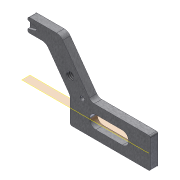
# Autodesk Inventor part: J002859
Saved by Autodesk Inventor 2012 SP2 (Build 160219200, 219)
## iProperties
Created: 2010-10-20
Part Number: J002859
Document SubType Name: Modeling
Designer: D Flickinger
Density: 8 g/cm^3
Material: STAINLESS STEEL, 303
Mass: 13.7432 g
Surface Area: 17.392 cm^2
Volume: 1.7179 cm^3
Description: MPS H Bar Clamp Bottom
Project: P-194005
Vendor: HHMI: JFRC - ID&F
d0: 1.150 in
d1: 1.200 in
d2: 0.575 in
d129: 0.00 deg
d132: 0.750 in
d136: 1.000 in
d137: 118.00 deg
d19: 0.125 in
d20: 0.00 deg
d21: 0.125 in
d22: 0.063 in
d23: 0.050 in
d24: 0.040 in
d25: 0.00 deg
d66: 0.125 in
d191: 0.000 in
ALTERED ITEM DESCRIPTION: N/A
ALTERED ITEM PART NUMBER: N/A
ALTERED ITEM VENDOR: N/A
DESIGN DEPARTMENT: HHMI: JFRC - ID&F
LAB/DEPT: SVOBODA (LAB)
REQUESTING SCIENTIST: PERON, SIMON
SPECIAL FINISH: NONE
SURFACE ROUGHNESS: 63 Ra
Revision Number: -
Autodesk Inventor part; units mm, degrees
ref_plane "YZ Plane" through (0, 0, 0) normal (1, 0, 0) x (0, 1, 0)
sketch "Sketch1" plane through (0, 0, 0) normal (0, 0, 1) x (1, 0, 0)
  line L0 (-20.447, 0) -> (20.447, 0) projected
  line L1 (0, -17.526) -> (0, 25.146) projected
  line L2 (14.605, -11.43) -> (-14.605, -11.43)
  line L3 (-14.605, -11.43) -> (-14.605, 19.05)
  line L4 (-14.605, 19.05) -> (14.605, 19.05)
  line L5 (14.605, 19.05) -> (14.605, -11.43)
  line L6 (-14.605, 16.6688) -> (-14.605, 19.05)
  point P0 (0, 0)
  dimension "d0" = 29.21
  dimension "d1" = 30.48
  dimension "d2" = 14.605
  dimension "d232" = 19.05
  constraints: 10 end point, 2 parallel, 1 collinear, 1 horizontal, 1 perpendicular, 1 point on line
  measures "d0" distance of L3.end L4.end
  measures "d1" distance of L2.end L3.end
  measures "d2" distance between parallel lines of L1 L3
  measures "d232" distance between parallel lines of L0 L4
extrude "Extrusion2" add sketch "Sketch1" along normal blind 3.175
sketch "Sketch2" plane through (0, 0, 3.175) normal (0, 0, 1) x (1, 0, 0)
  line L0 (-14.605, -11.43) -> (-14.605, 19.05) projected
  line L1 (-14.605, 17.78) -> (-11.43, 16.9862)
  line L2 (-11.43, 16.9862) -> (-11.43, 15.3987)
  line L3 (-11.43, 15.3987) -> (-14.605, 14.605)
  line L4 (-14.605, 17.78) -> (-14.605, 14.605)
  line L5 (-14.605, 17.78) -> (-14.605, 19.05)
  arc A0 (-11.43, 15.3987) -> (-11.43, 16.9862) centre (-11.6284, 16.1925) ccw
  point P0 (0, 0)
  dimension "d21" = 3.175
  dimension "d22" = 1.5875
  dimension "d23" = 1.27
  dimension "d66" = 3.175
  constraints: 10 end point, 2 collinear, 2 point on circle, 2 point on line, 1 centre point, 1 equal length, 1 parallel, 1 tangent
  measures "d21" distance of L1.start L3.end
  measures "d22" distance of L1.end L2.end
  measures "d23" distance of L1.start L0.end
  measures "d66" distance between parallel lines of L2 L0
extrude "Extrusion3" cut sketch "Sketch2" against normal blind 1.016
sketch "Sketch11" plane through (0, 0, 3.175) normal (0, 0, 1) x (1, 0, 0)
  line L0 (14.605, -11.43) -> (-14.605, -11.43) projected
  line L1 (14.605, 1.27) -> (14.605, 19.05)
  line L2 (-14.605, 13.335) -> (-6.985, 13.335)
  line L3 (-6.985, 13.335) -> (3.175, -0.8164)
  line L4 (10.795, -11.43) -> (-14.605, -11.43)
  line L5 (14.605, 19.05) -> (14.605, -11.43) projected
  line L6 (14.605, 1.27) -> (11.8393, 1.27)
  line L7 (11.8393, 1.27) -> (-0.9259, 19.05)
  line L8 (-0.9259, 19.05) -> (14.605, 19.05)
  line L9 (-14.605, 13.335) -> (-14.605, -11.43)
  line L10 (3.175, -0.8164) -> (3.175, -11.43)
  point P0 (0, 0)
  point P1 (0, -11.43)
  dimension "d220" = 7.62
  dimension "d221" = 25.4
  dimension "d226" = 12.7
  dimension "d230" = 8.255
  dimension "d263" = 7.62
  dimension "d264" = 54.324
  constraints: 18 end point, 4 perpendicular, 2 point on line, 1 midpoint, 1 parallel
  measures "d220" distance of L2.start L2.end
  measures "d221" distance of L4.start L0.end
  measures "d226" distance from line of L1.start L0
  measures "d230" distance between parallel lines of L7 L3
  measures "d263" distance of L4.start L10.end
  measures "d264" angle of L8 L7
extrude "Extrusion10" cut sketch "Sketch11" against normal through all
sketch "Sketch12" plane through (0, 0, 3.175) normal (0, 0, 1) x (1, 0, 0)
  line L0 (-14.605, 19.05) -> (14.605, 19.05) projected
  line L1 (-14.605, -11.43) -> (-14.605, 19.05) projected
  line L2 (-0.2249, 19.05) -> (-2.4073, 19.05)
  line L3 (-0.2419, 3.9428) -> (6.4638, 8.7572)
  line L4 (-0.2419, 3.9428) -> (3.111, 6.35)
  line L5 (3.111, 6.35) -> (6.4638, 8.7572)
  line L6 (-6.985, 13.335) -> (3.175, -0.8164) projected
  line L7 (11.8393, 1.27) -> (-0.9259, 19.05) projected
  line L8 (0, 25.146) -> (0, -17.526) projected
  line L9 (-20.447, 0) -> (20.447, 0) projected
  point P0 (-14.605, 14.605)
  point P1 (10.795, -11.43)
  dimension "d231" = 6.35
  constraints: 8 end point, 4 collinear, 2 perpendicular, 2 point on line, 1 midpoint, 1 other
hole "Hole9" at (3.111, 6.35, 3.175) direction (0, 0, -1) diameter 3.2512 end through all
sketch "Sketch16" plane through (14.605, -11.43, 3.175) normal (1, 0, 0) x (0, 0, -1)
  line L0 (3.175, 12.7) -> (0, 12.7) projected
  line L1 (0, 12.7) -> (0, 0) projected
  line L2 (3.175, 12.7) -> (3.175, 0) projected
  line L3 (3.175, 0) -> (0, 0) projected
  line L4 (0, 12.7) -> (3.175, 12.7)
  line L5 (3.175, 12.7) -> (3.175, 0)
  line L6 (3.175, 0) -> (0, 0)
  line L7 (0, 0) -> (0, 12.7)
  constraints: 8 end point, 2 parallel, 1 horizontal, 1 perpendicular
extrude "Extrusion14" add sketch "Sketch16" along normal blind 22.098
hole "Hole14-Orig threaded Tscrew hole" [suppressed]
sketch "Sketch17" plane through (0, 0, 0) normal (0, 0, 1) x (1, 0, 0)
  circle A0 centre (8.1788, 0.635) radius 0.7937
  circle A1 centre (3.111, 6.35) radius 1.6256 projected
  point P0 (0, 0)
  dimension "d235" = 1.5875
  dimension "d237" = 8.1788
  dimension "d238" = 5.0678
  dimension "d239" = 5.715
  constraints: 1 centre point
  measures "d235" diameter of A0
  measures "d237" horizontal distance of point (0, 0) A0.centre
  measures "d238" horizontal distance of A0.centre A1.centre
  measures "d239" vertical distance of A0.centre A1.centre
hole "Hole16" at (8.1788, 0.635, 0) direction (0, 0, 1) diameter 1.5748 end through all countersink diameter 1.905 countersink angle 90
fillet "Fillet9" radius 3.175 3 edges at (-0.9259, 19.05, 1.5875) (-6.985, 13.335, 1.5875) (3.175, -0.8164, 1.5875)
fillet "Fillet10" radius 0.635 2 edges at (-14.605, 19.05, 1.5875) (-14.605, 13.335, 1.5875)
ref_plane "Work Plane1" through (0, 0, 1.5875) normal (0, 0, 1) x (1, 0, 0)
mirror "Mirror1" about plane through (0, 0, 1.5875) normal (0, 0, 1) of "Extrusion3"
sketch "Sketch18" plane through (0, 0, 0) normal (0, 0, 1) x (1, 0, 0)
  line L0 (-13.97, 19.05) -> (-2.5549, 19.05) projected
  line L1 (-13.97, 13.335) -> (-8.6141, 13.335) projected
  line L2 (-14.605, 14.605) -> (-14.605, 17.78) projected
  line L3 (11.8393, 1.27) -> (0.0242, 17.7267) projected
  line L4 (-6.0349, 12.0117) -> (2.5791, 0.0135) projected
  circle A0 centre (3.111, 6.35) radius 1.6256 projected
  circle A1 centre (8.1788, 0.635) radius 0.7874 projected
  line L5 (-14.605, 19.05) -> (-0.9259, 19.05)
  line L6 (-6.985, 13.335) -> (-14.605, 13.335)
  line L7 (-14.605, 13.335) -> (-14.605, 19.05)
  line L8 (2.6983, -0.1524) -> (-6.985, 13.335)
  line L9 (-0.9259, 19.05) -> (7.3914, 7.4652)
  line L10 (7.3914, -0.1524) -> (2.6983, -0.1524)
  line L11 (7.3914, 7.4652) -> (7.3914, -0.1524)
  circle A2 centre (3.111, 6.35) radius 1.6256
  line L12 (-14.605, 17.78) -> (-14.605, 18.415) projected
  point P0 (10.8892, 2.5933)
  point P1 (9.8449, -10.1067)
  point P2 (10.795, -11.43)
  point P3 (6.985, -6.1232)
  dimension "d251" = 13.6791
  dimension "d252" = 5.715
  dimension "d253" = 7.62
  dimension "d254" = 14.2613
  dimension "d255" = 7.6176
  dimension "d256" = 4.6931
  dimension "d257" = 16.6035
  dimension "d258" = 21.9964
  dimension "d259" = 19.2024
  dimension "d260" = 12.7
  dimension "d261" = 17.716
  constraints: 14 end point, 4 collinear, 2 perpendicular, 2 point on line, 2 tangent, 1 centre point, 1 coincident, 1 concentric, 1 horizontal, 1 parallel, 1 vertical
  measures "d251" distance of L5.start L5.end
  measures "d252" distance of L6.end L5.start
  measures "d253" distance of L6.start L6.end
  measures "d254" distance of L5.end L9.end
  measures "d255" distance of L9.end L10.start
  measures "d256" distance of L10.start L8.start
  measures "d257" distance of L8.start L6.start
  measures "d258" distance between parallel lines of L11 L7
  measures "d259" distance between parallel lines of L10 L0
  measures "d260" distance from line of A0.centre L0
  measures "d261" distance from line of A0.centre L7
fillet "Fillet11" radius 0.635 3 edges at (36.703, -11.43, 1.5875) (36.703, 1.27, 1.5875) (3.175, -11.43, 1.5875)
fillet "Fillet12" radius 2.54 1 edges at (11.8393, 1.27, 1.5875)
sketch "Sketch19" plane through (0, 0, 0) normal (0, 0, 1) x (1, 0, 0)
  line L0 (11.303, -2.3495) -> (27.559, -2.3495)
  line L1 (27.559, -2.3495) -> (27.559, -7.8105)
  line L2 (27.559, -7.8105) -> (11.303, -7.8105)
  line L3 (11.303, -7.8105) -> (11.303, -2.3495)
  line L4 (27.559, -5.08) -> (11.303, -5.08) construction
  line L5 (19.431, -2.3495) -> (19.431, -7.8105) construction
  line L6 (36.703, -10.795) -> (36.703, 0.635) construction
  line L7 (36.068, -11.43) -> (3.81, -11.43) construction
  point P0 (0, 0)
  dimension "d267" = 16.256
  dimension "d268" = 5.461
  dimension "d269" = 6.35
  dimension "d274" = 19.431
  constraints: 12 end point, 4 midpoint, 2 parallel, 1 horizontal, 1 perpendicular
  measures "d267" distance of L0.start L0.end
  measures "d268" distance of L0.end L1.end
  measures "d269" distance between parallel lines of L7 L4
  measures "d274" distance from line of L5 point (0, 0)
extrude "Extrusion15" cut sketch "Sketch19" along normal through all
fillet "Fillet13" radius 2.54 4 edges at (11.303, -7.8105, 1.5875) (11.303, -2.3495, 1.5875) (27.559, -7.8105, 1.5875) (27.559, -2.3495, 1.5875)
ref_plane "Work Plane2" through (0, -5.0927, 0) normal (0, 1, 0) x (-1, 0, 0)
chamfer "Chamfer9" distance 0.1651 angle 45 1 edges at (8.1788, -0.1524, 3.175)
equation "\"d2\" = 0.5 * d0"
body "Solid2"
